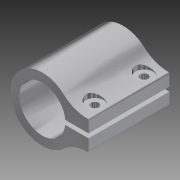
# Autodesk Inventor part: 739379
Saved by Autodesk Inventor 2018 (Build 220112000, 112)
## iProperties
Category: Fasteners
Company: Autodesk Inc.
Created: 2014-11-27
Part Number: 739379
Material: Aluminum 6061
Document SubType Name: Modeling
Designer: Tetrix
Density: 2.7 g/cm^3
Appearance: Aluminum - Polished
Vendor: Tetrix
Author: Autodesk Inc.
Autodesk Inventor part; units mm, degrees
ref_plane "XZ Plane" through (0, 0, 0) normal (0, 1, 0) x (-1, 0, 0)
ref_plane "XY Plane" through (0, 0, 0) normal (0, 0, 1) x (1, 0, 0)
sketch "Sketch1" plane through (0, 0, 0) normal (0, 1, 0) x (-1, 0, 0)
  line L0 (5, 15.5) -> (5, 15.4919)
  arc A0 (5, 15.5) -> (4.5, 16) centre (4.5, 15.5) ccw
  line L1 (0.75, 16) -> (4.5, 16)
  line L2 (0.75, 16) -> (0.75, 7.9145)
  arc A1 (-0.75, 7.9145) -> (0.75, 7.9145) centre (0, 0) ccw
  line L3 (-0.75, 7.9145) -> (-0.75, 16)
  line L4 (-4.5, 16) -> (-0.75, 16)
  arc A2 (-4.5, 16) -> (-5, 15.5) centre (-4.5, 15.5) ccw
  line L5 (-5, 15.4919) -> (-5, 15.5)
  arc A3 (-8.1304, 7.4092) -> (-5, 15.4919) centre (-17, 15.4919) ccw
  arc A4 (-8.1304, 7.4092) -> (8.1304, 7.4092) centre (0, 0) ccw
  arc A5 (5, 15.4919) -> (8.1304, 7.4092) centre (17, 15.4919) ccw
  constraints: 12 end point, 12 point on circle, 6 centre point
extrude "Extrusion1" add sketch "Sketch1" against normal blind 28
ref_plane "Work Plane1" through (-11, 0, 0) normal (1, 0, 0) x (0, 1, 0)
sketch "Sketch2" plane through (-11, 0, 0) normal (1, 0, 0) x (0, 1, 0)
  line L0 (-28, 7.4092) -> (-28, 15.4919) projected
  line L1 (0, 15.4919) -> (0, 7.4092) projected
  line L2 (0, 16) -> (-28, 16) projected
  circle A0 centre (-22.4133, 12.6) radius 1.35
  circle A1 centre (-5.3496, 12.6) radius 1.35
  circle A2 centre (-22.4133, 12.6) radius 3
  circle A3 centre (-5.3496, 12.6) radius 3
  point P0 (0, 0)
  dimension "d2" = 3.4
  dimension "d3" = 2.7
  dimension "d4" = 2.7
  dimension "d7" = 6
  constraints: 4 centre point, 4 coincident, 1 equal radius, 1 horizontal alignment
  measures "d2" distance from line of point (-22.413, 12.6) L2
  measures "d3" diameter of A0
  measures "d4" diameter of A1
  measures "d7" diameter of A2
extrude "Extrusion2" cut sketch "Sketch2" along normal up to surface contours A0 | A1 round surface about axis through (17, 0, 15.4919) along (0, -1, 0) radius 12 far side no
extrude "Extrusion3" cut sketch "Sketch2" along normal blind 6.25
thread "Thread1" size "M3x0.5" class "6H" standard "ANSI Metric M Profile" full length
thread "Thread2" size "M3x0.5" class "6H" standard "ANSI Metric M Profile" full length
body "Solid1"
